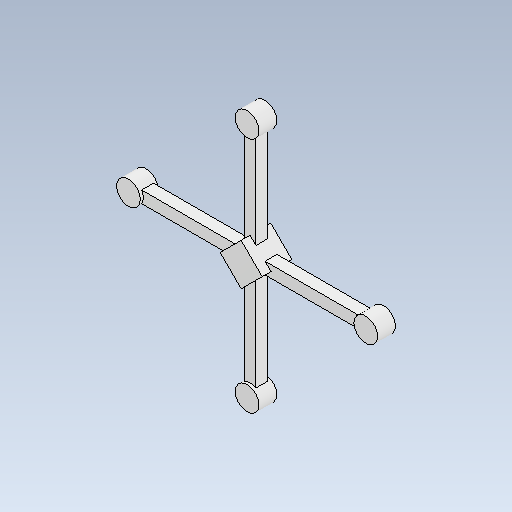
# Autodesk Inventor part: drohne_model
Saved by Autodesk Inventor 2025 (Build 290162000, 162)
## iProperties
Created: 2026-04-25
Part Number: drohne_model
Material: PC/ABS-Kunststoff
Document SubType Name: Modeling
Designer: andit
Density: 1.1 g/cm^3
Appearance: Glatt - Weiß
Mass: 568.278 g
Surface Area: 854.483 cm^2
Volume: 516.616 cm^3
Author: andit
Autodesk Inventor part; units mm, degrees
ref_plane "YZ Plane" through (0, 0, 0) normal (1, 0, 0) x (0, 1, 0)
ref_plane "XZ Plane" through (0, 0, 0) normal (0, 1, 0) x (-1, 0, 0)
ref_plane "XY Plane" through (0, 0, 0) normal (0, 0, 1) x (1, 0, 0)
sketch "Skizze1" plane through (0, 0, 0) normal (0, 0, 1) x (1, 0, 0)
  line L0 (-35.3553, 0) -> (0, 35.3553)
  line L1 (0, 35.3553) -> (35.3553, 0)
  line L2 (35.3553, 0) -> (0, -35.3553)
  line L3 (0, -35.3553) -> (-35.3553, 0)
  line L4 (-35.3553, 0) -> (35.3553, 0) construction
  line L5 (0, 35.3553) -> (0, -35.3553) construction
  point P0 (0, 0)
  point P1 (0, 0)
  dimension "d0" = 50
  dimension "d1" = 50
  constraints: 12 end point, 3 midpoint, 2 parallel, 1 perpendicular, 1 vertical alignment
  measures "d0" distance of L0.end L1.end
  measures "d1" distance of L0.start L0.end
extrude "Extrusion1" add sketch "Skizze1" along normal mid plane 50
sketch "Skizze2" plane through (0, 0, 0) normal (0, 0, 1) x (1, 0, 0)
  line L0 (-200, 10) -> (200, 10)
  line L1 (200, 10) -> (200, -10)
  line L2 (200, -10) -> (-200, -10)
  line L3 (-200, -10) -> (-200, 10)
  line L4 (-200, 10) -> (200, -10) construction
  line L5 (200, 10) -> (-200, -10) construction
  line L6 (-10, -200) -> (-10, 200)
  line L7 (-10, 200) -> (10, 200)
  line L8 (10, 200) -> (10, -200)
  line L9 (10, -200) -> (-10, -200)
  point P0 (0, 0)
  point P1 (0, 200)
  point P2 (-10, 0)
  point P3 (0, -200)
  point P4 (-10, -10)
  point P5 (10, -10)
  point P6 (10, 10)
  point P7 (-10, 10)
  dimension "d4" = 400
  dimension "d5" = 20
  dimension "d6" = 400
  dimension "d7" = 20
  constraints: 20 end point, 5 midpoint, 4 parallel, 2 perpendicular, 2 vertical alignment, 1 horizontal, 1 horizontal alignment
  measures "d4" distance of L1.end L2.end
  measures "d5" distance of L0.end L1.end
  measures "d6" distance of L8.start L9.start
  measures "d7" distance of L6.end L8.start
extrude "Extrusion2" add sketch "Skizze2" along normal mid plane 20
sketch "Skizze3" plane through (0, 0, 0) normal (0, 0, 1) x (1, 0, 0)
  line L0 (-200, -10) -> (-200, 10) projected
  circle A0 centre (-200, 0) radius 20
  circle A1 centre (0, -200) radius 20
  circle A2 centre (200, 0) radius 20
  circle A3 centre (0, 200) radius 20
  point P0 (0, 0)
  dimension "d10" = 40
  dimension "d13" = 360
  constraints: 4 centre point, 1 midpoint, 9 other
  measures "d10" diameter of A0
extrude "Extrusion3" add sketch "Skizze3" along normal mid plane 30
